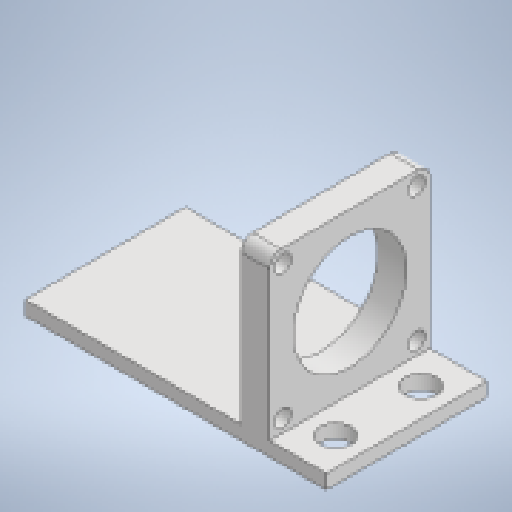
# Autodesk Inventor part: NEMA23_Mount
Saved by Autodesk Inventor 2023 (Build 270158000, 158)
## iProperties
Created: 2022-04-30
Part Number: NEMA23_Mount
Material: Generic
Document SubType Name: Modeling
Designer: plebbb
Density: 1 g/cm^3
Appearance: Default
Author: plebbb
Autodesk Inventor part; units mm, degrees
ref_plane "YZ Plane" through (0, 0, 0) normal (1, 0, 0) x (0, 1, 0)
ref_plane "XZ Plane" through (0, 0, 0) normal (0, 1, 0) x (-1, 0, 0)
ref_plane "XY Plane" through (0, 0, 0) normal (0, 0, 1) x (1, 0, 0)
sketch "Sketch1" plane through (0, 0, 0) normal (1, 0, 0) x (0, 1, 0)
  line L0 (56.4, 0) -> (0, 0)
  line L1 (0, 0) -> (0, -56.4)
  line L2 (0, -56.4) -> (56.4, -56.4)
  line L3 (56.4, -56.4) -> (56.4, 0)
  line L4 (51.77, -4.63) -> (4.63, -4.63) construction
  line L5 (4.63, -4.63) -> (4.63, -51.77) construction
  line L6 (4.63, -51.77) -> (51.77, -51.77) construction
  line L7 (51.77, -51.77) -> (51.77, -4.63) construction
  circle A0 centre (28.2, -28.2) radius 20
  circle A1 centre (51.77, -4.63) radius 3
  circle A2 centre (51.77, -51.77) radius 3
  circle A3 centre (4.63, -4.63) radius 3
  circle A4 centre (4.63, -51.77) radius 3
  arc A5 (56.4, -4) -> (52.4, 0) centre (52.4, -4) ccw
  arc A6 (52.4, -56.4) -> (56.4, -52.4) centre (52.4, -52.4) ccw
  point P0 (51.77, -28.2)
  point P1 (56.4, -28.2)
  point P2 (28.2, -56.4)
  point P3 (28.2, -51.77)
  dimension "d0" = 56.4
  dimension "d1" = 47.14
  dimension "d2" = 40
  dimension "d3" = 6
  dimension "d4" = 4
  dimension "d5" = 4
  constraints: 16 end point, 7 centre point, 5 coincident, 4 midpoint, 4 parallel, 4 perpendicular, 4 point on circle, 4 point on line, 4 tangent, 3 equal radius, 2 horizontal, 2 horizontal alignment, 2 vertical alignment
  measures "d0" distance of L2.end L0.start
  measures "d1" distance of L6.end L4.start
  measures "d2" diameter of A0
  measures "d3" diameter of A1
  measures "d4" radius of A5
  measures "d5" radius of A6
extrude "Extrusion1" add sketch "Sketch1" along normal blind 10 contours A5 L3 A6 L2 L1 L0
sketch "Sketch2" plane through (0, 0, -56.4) normal (0, -1, 0) x (1, 0, 0)
  line L0 (-76, 0) -> (30, 0)
  line L1 (30, 0) -> (30, 56.4)
  line L2 (30, 56.4) -> (-76, 56.4)
  line L3 (-76, 56.4) -> (-76, 0)
  circle A0 centre (20, 43.2) radius 5.5
  circle A1 centre (20, 13.2) radius 5.5
  line L4 (20, 43.2) -> (20, 13.2) construction
  line L5 (10, 56.4) -> (20, 43.2) construction
  line L6 (30, 56.4) -> (20, 43.2) construction
  point P0 (0, 56.4)
  point P1 (0, 0)
  point P2 (20, 28.2)
  point P3 (30, 28.2)
  dimension "d8" = 30
  dimension "d9" = 76
  dimension "d10" = 11
  dimension "d11" = 11
  dimension "d12" = 30
  constraints: 14 end point, 2 centre point, 2 midpoint, 2 parallel, 2 point on line, 1 equal length, 1 horizontal, 1 horizontal alignment, 1 perpendicular, 1 vertical, 1 vertical alignment
  measures "d8" distance from line of point (0, 56.4) L1
  measures "d9" distance of L2.end point (0, 56.4)
  measures "d10" diameter of A0
  measures "d11" diameter of A1
  measures "d12" distance of L4.end L4.start
extrude "Extrusion2" add sketch "Sketch2" along normal blind 5
body "Solid1"
